Autodesk Fusion 360 part; units mm, degrees
(part 8 of 15)
  spline S16 degree 5 poles (-0.9615, -15.0052) (-0.9615, -15.0053) (-0.9615, -15.0055) (-0.9615, -15.0058) (-0.9616, -15.0063) (-0.9616, -15.0071) (-0.9616, -15.008) (-0.9617, -15.0091) (-0.9617, -15.0102) (-0.9618, -15.0115) (-0.9618, -15.0128) (-0.9619, -15.0143) (-0.9619, -15.0159) (-0.9619, -15.0176) (-0.962, -15.0194) (-0.962, -15.0213) (-0.962, -15.0234) (-0.9621, -15.0255) (-0.9621, -15.0277) (-0.9621, -15.0301) (-0.9621, -15.0325) (-0.9621, -15.0351) (-0.9621, -15.0377) (-0.9621, -15.0404) (-0.9621, -15.0433) (-0.9621, -15.0462) (-0.962, -15.0492) (-0.962, -15.0523) (-0.9619, -15.0555) (-0.9619, -15.0588) (-0.9618, -15.0622) (-0.9617, -15.0657) (-0.9616, -15.0693) (-0.9615, -15.0729) (-0.9614, -15.0767) (-0.9612, -15.0805) (-0.9611, -15.0844) (-0.9609, -15.0884) (-0.9607, -15.0925) (-0.9606, -15.0967) (-0.9603, -15.1009) (-0.9601, -15.1053) (-0.9599, -15.1097) (-0.9596, -15.1142) (-0.9594, -15.1187) (-0.9591, -15.1234) (-0.9588, -15.1281) (-0.9585, -15.1329) (-0.9581, -15.1378) (-0.9578, -15.1427) (-0.9574, -15.1477) (-0.957, -15.1528) (-0.9566, -15.158) (-0.9562, -15.1633) (-0.9558, -15.1686) (-0.9553, -15.174) (-0.9548, -15.1794) (-0.9543, -15.1849) (-0.9538, -15.1905) (-0.9533, -15.1962) (-0.9527, -15.2019) (-0.9521, -15.2077) (-0.9515, -15.2136) (-0.9509, -15.2196) (-0.9503, -15.2256) (-0.9496, -15.2316) (-0.9489, -15.2378) (-0.9482, -15.244) (-0.9475, -15.2502) (-0.9467, -15.2565) (-0.946, -15.2629) (-0.9452, -15.2694) (-0.9444, -15.2759) (-0.9435, -15.2825) (-0.9427, -15.2891) (-0.9418, -15.2958) (-0.9408, -15.3025) (-0.9399, -15.3094) (-0.9389, -15.3162) (-0.938, -15.3232) (-0.937, -15.3301) (-0.9359, -15.3372) (-0.9349, -15.3443) (-0.9338, -15.3515) (-0.9327, -15.3587) (-0.9315, -15.3659) (-0.9304, -15.3733) (-0.9292, -15.3807) (-0.928, -15.3881) (-0.9267, -15.3956) (-0.9255, -15.4031) (-0.9242, -15.4107) (-0.9229, -15.4184) (-0.9215, -15.4261) (-0.9202, -15.4338) (-0.9188, -15.4417) (-0.9173, -15.4495) (-0.9159, -15.4574) (-0.9144, -15.4654) (-0.9129, -15.4734) (-0.9114, -15.4815) (-0.9098, -15.4896) (-0.9082, -15.4977) (-0.9066, -15.5059) (-0.905, -15.5142) (-0.9033, -15.5225) (-0.9016, -15.5309) (-0.8999, -15.5393) (-0.8981, -15.5477) (-0.8963, -15.5562) (-0.8945, -15.5648) (-0.8927, -15.5733) (-0.8908, -15.582) (-0.8889, -15.5907) (-0.887, -15.5994) (-0.885, -15.6081) (-0.883, -15.617) (-0.881, -15.6258) (-0.879, -15.6347) (-0.8769, -15.6437) (-0.8748, -15.6527) (-0.8726, -15.6617) (-0.8705, -15.6708) (-0.8683, -15.6799) (-0.866, -15.689) (-0.8638, -15.6982) (-0.8615, -15.7075) (-0.8592, -15.7168) (-0.8568, -15.7261) (-0.8544, -15.7354) (-0.852, -15.7448) (-0.8496, -15.7543) (-0.8471, -15.7638) (-0.8446, -15.7733) (-0.8421, -15.7829) (-0.8395, -15.7925) (-0.8369, -15.8021) (-0.8343, -15.8118) (-0.8316, -15.8215) (-0.8289, -15.8313) (-0.8262, -15.841) (-0.8235, -15.8509) (-0.8207, -15.8607) (-0.8178, -15.8706) (-0.815, -15.8806) (-0.8121, -15.8906) (-0.8092, -15.9006) (-0.8063, -15.9106) (-0.8033, -15.9207) (-0.8003, -15.9308) (-0.7972, -15.941) (-0.7941, -15.9512) (-0.791, -15.9614) (-0.7879, -15.9716) (-0.7847, -15.9819) (-0.7815, -15.9923) (-0.7783, -16.0026) (-0.775, -16.013) (-0.7717, -16.0234) (-0.7683, -16.0339) (-0.765, -16.0444) (-0.7616, -16.0549) (-0.7581, -16.0655) (-0.7547, -16.0761) (-0.7512, -16.0867) (-0.7476, -16.0973) (-0.744, -16.108) (-0.7404, -16.1187) (-0.7368, -16.1295) (-0.7331, -16.1402) (-0.7294, -16.151) (-0.7257, -16.1619) (-0.7219, -16.1727) (-0.7181, -16.1836) (-0.7143, -16.1946) (-0.7104, -16.2055) (-0.7065, -16.2165) (-0.7025, -16.2275) (-0.6986, -16.2385) (-0.6946, -16.2496) (-0.6905, -16.2607) (-0.6864, -16.2718) (-0.6823, -16.283) (-0.6782, -16.2942) (-0.674, -16.3054) (-0.6698, -16.3166) (-0.6655, -16.3279) (-0.6612, -16.3391) (-0.6569, -16.3505) (-0.6526, -16.3618) (-0.6482, -16.3732) (-0.6438, -16.3846) (-0.6393, -16.396) (-0.6348, -16.4074) (-0.6303, -16.4189) (-0.6257, -16.4304) (-0.6211, -16.4419) (-0.6165, -16.4535) (-0.6118, -16.465) (-0.6071, -16.4766) (-0.6024, -16.4882) (-0.5976, -16.4999) (-0.5928, -16.5116) (-0.588, -16.5233) (-0.5831, -16.535) (-0.5782, -16.5467) (-0.5732, -16.5585) (-0.5683, -16.5703) (-0.5632, -16.5821) (-0.5582, -16.5939) (-0.5531, -16.6057) (-0.548, -16.6176) (-0.5428, -16.6295) (-0.5376, -16.6414) (-0.5324, -16.6534) (-0.5271, -16.6653) (-0.5218, -16.6773) (-0.5165, -16.6893) (-0.5111, -16.7014) (-0.5057, -16.7134) (-0.5003, -16.7255) (-0.4948, -16.7376) (-0.4893, -16.7497) (-0.4837, -16.7618) (-0.4782, -16.774) (-0.4725, -16.7861) (-0.4669, -16.7983) (-0.4612, -16.8105) (-0.4555, -16.8228) (-0.4497, -16.835) (-0.4439, -16.8473) (-0.4381, -16.8596) (-0.4322, -16.8719) (-0.4263, -16.8842) (-0.4203, -16.8965) (-0.4144, -16.9089) (-0.4084, -16.9213) (-0.4023, -16.9337) (-0.3962, -16.9461) (-0.3901, -16.9585) (-0.3839, -16.971) (-0.379, -16.981) (-0.3753, -16.9884) (-0.3728, -16.9934) (-0.3715, -16.9959) knots 0 0 0 0 0 0 0.00416667 0.00833333 0.0125 0.01666667 0.02083333 0.025 0.02916667 0.03333333 0.0375 0.04166667 0.04583333 0.05 0.05416667 0.05833333 0.0625 0.06666667 0.07083333 0.075 0.07916667 0.08333333 0.0875 0.09166667 0.09583333 0.1 0.10416667 0.10833333 0.1125 0.11666667 0.12083333 0.125 0.12916667 0.13333333 0.1375 0.14166667 0.14583333 0.15 0.15416667 0.15833333 0.1625 0.16666667 0.17083333 0.175 0.17916667 0.18333333 0.1875 0.19166667 0.19583333 0.2 0.20416667 0.20833333 0.2125 0.21666667 0.22083333 0.225 0.22916667 0.23333333 0.2375 0.24166667 0.24583333 0.25 0.25416667 0.25833333 0.2625 0.26666667 0.27083333 0.275 0.27916667 0.28333333 0.2875 0.29166667 0.29583333 0.3 0.30416667 0.30833333 0.3125 0.31666667 0.32083333 0.325 0.32916667 0.33333333 0.3375 0.34166667 0.34583333 0.35 0.35416667 0.35833333 0.3625 0.36666667 0.37083333 0.375 0.37916667 0.38333333 0.3875 0.39166667 0.39583333 0.4 0.40416667 0.40833333 0.4125 0.41666667 0.42083333 0.425 0.42916667 0.43333333 0.4375 0.44166667 0.44583333 0.45 0.45416667 0.45833333 0.4625 0.46666667 0.47083333 0.475 0.47916667 0.48333333 0.4875 0.49166667 0.49583333 0.5 0.50416667 0.50833333 0.5125 0.51666667 0.52083333 0.525 0.52916667 0.53333333 0.5375 0.54166667 0.54583333 0.55 0.55416667 0.55833333 0.5625 0.56666667 0.57083333 0.575 0.57916667 0.58333333 0.5875 0.59166667 0.59583333 0.6 0.60416667 0.60833333 0.6125 0.61666667 0.62083333 0.625 0.62916667 0.63333333 0.6375 0.64166667 0.64583333 0.65 0.65416667 0.65833333 0.6625 0.66666667 0.67083333 0.675 0.67916667 0.68333333 0.6875 0.69166667 0.69583333 0.7 0.70416667 0.70833333 0.7125 0.71666667 0.72083333 0.725 0.72916667 0.73333333 0.7375 0.74166667 0.74583333 0.75 0.75416667 0.75833333 0.7625 0.76666667 0.77083333 0.775 0.77916667 0.78333333 0.7875 0.79166667 0.79583333 0.8 0.80416667 0.80833333 0.8125 0.81666667 0.82083333 0.825 0.82916667 0.83333333 0.8375 0.84166667 0.84583333 0.85 0.85416667 0.85833333 0.8625 0.86666667 0.87083333 0.875 0.87916667 0.88333333 0.8875 0.89166667 0.89583333 0.9 0.90416667 0.90833333 0.9125 0.91666667 0.92083333 0.925 0.92916667 0.93333333 0.9375 0.94166667 0.94583333 0.95 0.95416667 0.95833333 0.9625 0.96666667 0.97083333 0.975 0.97916667 0.98333333 0.9875 0.99166667 0.99583333 1 1 1 1 1 1
  arc A17 (-0.3715, -16.9959) -> (0.3715, -16.9959) centre (0, 0) ccw
  spline S17 degree 5 poles (0.3715, -16.9959) (0.3728, -16.9934) (0.3753, -16.9884) (0.379, -16.981) (0.3839, -16.971) (0.3901, -16.9585) (0.3962, -16.9461) (0.4023, -16.9337) (0.4084, -16.9213) (0.4144, -16.9089) (0.4203, -16.8965) (0.4263, -16.8842) (0.4322, -16.8719) (0.4381, -16.8596) (0.4439, -16.8473) (0.4497, -16.835) (0.4555, -16.8228) (0.4612, -16.8105) (0.4669, -16.7983) (0.4725, -16.7861) (0.4782, -16.774) (0.4837, -16.7618) (0.4893, -16.7497) (0.4948, -16.7376) (0.5003, -16.7255) (0.5057, -16.7134) (0.5111, -16.7014) (0.5165, -16.6893) (0.5218, -16.6773) (0.5271, -16.6653) (0.5324, -16.6534) (0.5376, -16.6414) (0.5428, -16.6295) (0.548, -16.6176) (0.5531, -16.6057) (0.5582, -16.5939) (0.5632, -16.5821) (0.5683, -16.5703) (0.5732, -16.5585) (0.5782, -16.5467) (0.5831, -16.535) (0.588, -16.5233) (0.5928, -16.5116) (0.5976, -16.4999) (0.6024, -16.4882) (0.6071, -16.4766) (0.6118, -16.465) (0.6165, -16.4535) (0.6211, -16.4419) (0.6257, -16.4304) (0.6303, -16.4189) (0.6348, -16.4074) (0.6393, -16.396) (0.6438, -16.3846) (0.6482, -16.3732) (0.6526, -16.3618) (0.6569, -16.3505) (0.6612, -16.3391) (0.6655, -16.3279) (0.6698, -16.3166) (0.674, -16.3054) (0.6782, -16.2942) (0.6823, -16.283) (0.6864, -16.2718) (0.6905, -16.2607) (0.6946, -16.2496) (0.6986, -16.2385) (0.7025, -16.2275) (0.7065, -16.2165) (0.7104, -16.2055) (0.7143, -16.1946) (0.7181, -16.1836) (0.7219, -16.1727) (0.7257, -16.1619) (0.7294, -16.151) (0.7331, -16.1402) (0.7368, -16.1295) (0.7404, -16.1187) (0.744, -16.108) (0.7476, -16.0973) (0.7512, -16.0867) (0.7547, -16.0761) (0.7581, -16.0655) (0.7616, -16.0549) (0.765, -16.0444) (0.7683, -16.0339) (0.7717, -16.0234) (0.775, -16.013) (0.7783, -16.0026) (0.7815, -15.9923) (0.7847, -15.9819) (0.7879, -15.9716) (0.791, -15.9614) (0.7941, -15.9512) (0.7972, -15.941) (0.8003, -15.9308) (0.8033, -15.9207) (0.8063, -15.9106) (0.8092, -15.9006) (0.8121, -15.8906) (0.815, -15.8806) (0.8178, -15.8706) (0.8207, -15.8607) (0.8235, -15.8509) (0.8262, -15.841) (0.8289, -15.8313) (0.8316, -15.8215) (0.8343, -15.8118) (0.8369, -15.8021) (0.8395, -15.7925) (0.8421, -15.7829) (0.8446, -15.7733) (0.8471, -15.7638) (0.8496, -15.7543) (0.852, -15.7448) (0.8544, -15.7354) (0.8568, -15.7261) (0.8592, -15.7168) (0.8615, -15.7075) (0.8638, -15.6982) (0.866, -15.689) (0.8683, -15.6799) (0.8705, -15.6708) (0.8726, -15.6617) (0.8748, -15.6527) (0.8769, -15.6437) (0.879, -15.6347) (0.881, -15.6258) (0.883, -15.617) (0.885, -15.6081) (0.887, -15.5994) (0.8889, -15.5907) (0.8908, -15.582) (0.8927, -15.5733) (0.8945, -15.5648) (0.8963, -15.5562) (0.8981, -15.5477) (0.8999, -15.5393) (0.9016, -15.5309) (0.9033, -15.5225) (0.905, -15.5142) (0.9066, -15.5059) (0.9082, -15.4977) (0.9098, -15.4896) (0.9114, -15.4815) (0.9129, -15.4734) (0.9144, -15.4654) (0.9159, -15.4574) (0.9173, -15.4495) (0.9188, -15.4417) (0.9202, -15.4338) (0.9215, -15.4261) (0.9229, -15.4184) (0.9242, -15.4107) (0.9255, -15.4031) (0.9267, -15.3956) (0.928, -15.3881) (0.9292, -15.3807) (0.9304, -15.3733) (0.9315, -15.3659) (0.9327, -15.3587) (0.9338, -15.3515) (0.9349, -15.3443) (0.9359, -15.3372) (0.937, -15.3301) (0.938, -15.3232) (0.9389, -15.3162) (0.9399, -15.3094) (0.9408, -15.3025) (0.9418, -15.2958) (0.9427, -15.2891) (0.9435, -15.2825) (0.9444, -15.2759) (0.9452, -15.2694) (0.946, -15.2629) (0.9467, -15.2565) (0.9475, -15.2502) (0.9482, -15.244) (0.9489, -15.2378) (0.9496, -15.2316) (0.9503, -15.2256) (0.9509, -15.2196) (0.9515, -15.2136) (0.9521, -15.2077) (0.9527, -15.2019) (0.9533, -15.1962) (0.9538, -15.1905) (0.9543, -15.1849) (0.9548, -15.1794) (0.9553, -15.174) (0.9558, -15.1686) (0.9562, -15.1633) (0.9566, -15.158) (0.957, -15.1528) (0.9574, -15.1477) (0.9578, -15.1427) (0.9581, -15.1378) (0.9585, -15.1329) (0.9588, -15.1281) (0.9591, -15.1234) (0.9594, -15.1187) (0.9596, -15.1142) (0.9599, -15.1097) (0.9601, -15.1053) (0.9603, -15.1009) (0.9606, -15.0967) (0.9607, -15.0925) (0.9609, -15.0884) (0.9611, -15.0844) (0.9612, -15.0805) (0.9614, -15.0767) (0.9615, -15.0729) (0.9616, -15.0693) (0.9617, -15.0657) (0.9618, -15.0622) (0.9619, -15.0588) (0.9619, -15.0555) (0.962, -15.0523) (0.962, -15.0492) (0.9621, -15.0462) (0.9621, -15.0433) (0.9621, -15.0404) (0.9621, -15.0377) (0.9621, -15.0351) (0.9621, -15.0325) (0.9621, -15.0301) (0.9621, -15.0277) (0.9621, -15.0255) (0.962, -15.0234) (0.962, -15.0213) (0.962, -15.0194) (0.9619, -15.0176) (0.9619, -15.0159) (0.9619, -15.0143) (0.9618, -15.0128) (0.9618, -15.0115) (0.9617, -15.0102) (0.9617, -15.0091) (0.9616, -15.008) (0.9616, -15.0071) (0.9616, -15.0063) (0.9615, -15.0058) (0.9615, -15.0055) (0.9615, -15.0053) (0.9615, -15.0052) knots -1 -1 -1 -1 -1 -1 -0.99583333 -0.99166667 -0.9875 -0.98333333 -0.97916667 -0.975 -0.97083333 -0.96666667 -0.9625 -0.95833333 -0.95416667 -0.95 -0.94583333 -0.94166667 -0.9375 -0.93333333 -0.92916667 -0.925 -0.92083333 -0.91666667 -0.9125 -0.90833333 -0.90416667 -0.9 -0.89583333 -0.89166667 -0.8875 -0.88333333 -0.87916667 -0.875 -0.87083333 -0.86666667 -0.8625 -0.85833333 -0.85416667 -0.85 -0.84583333 -0.84166667 -0.8375 -0.83333333 -0.82916667 -0.825 -0.82083333 -0.81666667 -0.8125 -0.80833333 -0.80416667 -0.8 -0.79583333 -0.79166667 -0.7875 -0.78333333 -0.77916667 -0.775 -0.77083333 -0.76666667 -0.7625 -0.75833333 -0.75416667 -0.75 -0.74583333 -0.74166667 -0.7375 -0.73333333 -0.72916667 -0.725 -0.72083333 -0.71666667 -0.7125 -0.70833333 -0.70416667 -0.7 -0.69583333 -0.69166667 -0.6875 -0.68333333 -0.67916667 -0.675 -0.67083333 -0.66666667 -0.6625 -0.65833333 -0.65416667 -0.65 -0.64583333 -0.64166667 -0.6375 -0.63333333 -0.62916667 -0.625 -0.62083333 -0.61666667 -0.6125 -0.60833333 -0.60416667 -0.6 -0.59583333 -0.59166667 -0.5875 -0.58333333 -0.57916667 -0.575 -0.57083333 -0.56666667 -0.5625 -0.55833333 -0.55416667 -0.55 -0.54583333 -0.54166667 -0.5375 -0.53333333 -0.52916667 -0.525 -0.52083333 -0.51666667 -0.5125 -0.50833333 -0.50416667 -0.5 -0.49583333 -0.49166667 -0.4875 -0.48333333 -0.47916667 -0.475 -0.47083333 -0.46666667 -0.4625 -0.45833333 -0.45416667 -0.45 -0.44583333 -0.44166667 -0.4375 -0.43333333 -0.42916667 -0.425 -0.42083333 -0.41666667 -0.4125 -0.40833333 -0.40416667 -0.4 -0.39583333 -0.39166667 -0.3875 -0.38333333 -0.37916667 -0.375 -0.37083333 -0.36666667 -0.3625 -0.35833333 -0.35416667 -0.35 -0.34583333 -0.34166667 -0.3375 -0.33333333 -0.32916667 -0.325 -0.32083333 -0.31666667 -0.3125 -0.30833333 -0.30416667 -0.3 -0.29583333 -0.29166667 -0.2875 -0.28333333 -0.27916667 -0.275 -0.27083333 -0.26666667 -0.2625 -0.25833333 -0.25416667 -0.25 -0.24583333 -0.24166667 -0.2375 -0.23333333 -0.22916667 -0.225 -0.22083333 -0.21666667 -0.2125 -0.20833333 -0.20416667 -0.2 -0.19583333 -0.19166667 -0.1875 -0.18333333 -0.17916667 -0.175 -0.17083333 -0.16666667 -0.1625 -0.15833333 -0.15416667 -0.15 -0.14583333 -0.14166667 -0.1375 -0.13333333 -0.12916667 -0.125 -0.12083333 -0.11666667 -0.1125 -0.10833333 -0.10416667 -0.1 -0.09583333 -0.09166667 -0.0875 -0.08333333 -0.07916667 -0.075 -0.07083333 -0.06666667 -0.0625 -0.05833333 -0.05416667 -0.05 -0.04583333 -0.04166667 -0.0375 -0.03333333 -0.02916667 -0.025 -0.02083333 -0.01666667 -0.0125 -0.00833333 -0.00416667 0 0 0 0 0 0
  line L34 (0.9615, -15.0052) -> (0.9615, -15.0043)
  line L35 (0.9615, -15.0043) -> (0.9432, -14.7198)
  arc A18 (0.9432, -14.7198) -> (1.9466, -14.621) centre (0, 0) ccw
  line L36 (1.9466, -14.621) -> (1.9842, -14.9036)
  line L37 (1.9842, -14.9036) -> (1.9843, -14.9044)
  spline S18 degree 5 poles (1.9843, -14.9044) (1.9843, -14.9045) (1.9844, -14.9047) (1.9844, -14.9051) (1.9845, -14.9056) (1.9846, -14.9064) (1.9848, -14.9073) (1.9849, -14.9083) (1.9851, -14.9094) (1.9853, -14.9106) (1.9855, -14.912) (1.9858, -14.9135) (1.986, -14.915) (1.9863, -14.9167) (1.9866, -14.9185) (1.987, -14.9204) (1.9874, -14.9224) (1.9877, -14.9245) (1.9882, -14.9267) (1.9886, -14.929) (1.9891, -14.9314) (1.9896, -14.9339) (1.9901, -14.9365) (1.9906, -14.9391) (1.9912, -14.9419) (1.9918, -14.9448) (1.9924, -14.9477) (1.9931, -14.9508) (1.9937, -14.9539) (1.9945, -14.9571) (1.9952, -14.9605) (1.996, -14.9639) (1.9968, -14.9673) (1.9976, -14.9709) (1.9984, -14.9746) (1.9993, -14.9783) (2.0002, -14.9821) (2.0012, -14.986) (2.0021, -14.99) (2.0031, -14.994) (2.0042, -14.9981) (2.0052, -15.0023) (2.0063, -15.0066) (2.0074, -15.011) (2.0086, -15.0154) (2.0098, -15.0199) (2.011, -15.0245) (2.0122, -15.0291) (2.0135, -15.0338) (2.0148, -15.0386) (2.0161, -15.0435) (2.0175, -15.0484) (2.0189, -15.0534) (2.0204, -15.0584) (2.0218, -15.0636) (2.0233, -15.0688) (2.0249, -15.074) (2.0264, -15.0794) (2.028, -15.0847) (2.0297, -15.0902) (2.0313, -15.0957) (2.033, -15.1013) (2.0348, -15.1069) (2.0365, -15.1126) (2.0383, -15.1184) (2.0402, -15.1242) (2.042, -15.1301) (2.0439, -15.136) (2.0459, -15.142) (2.0478, -15.1481) (2.0499, -15.1542) (2.0519, -15.1604) (2.054, -15.1666) (2.0561, -15.1729) (2.0582, -15.1792) (2.0604, -15.1856) (2.0626, -15.1921) (2.0649, -15.1986) (2.0671, -15.2051) (2.0695, -15.2117) (2.0718, -15.2184) (2.0742, -15.2251) (2.0766, -15.2318) (2.0791, -15.2387) (2.0816, -15.2455) (2.0841, -15.2524) (2.0867, -15.2594) (2.0893, -15.2664) (2.0919, -15.2735) (2.0946, -15.2806) (2.0973, -15.2877) (2.1001, -15.2949) (2.1028, -15.3022) (2.1057, -15.3095) (2.1085, -15.3168) (2.1114, -15.3242) (2.1143, -15.3316) (2.1173, -15.3391) (2.1203, -15.3466) (2.1233, -15.3542) (2.1264, -15.3618) (2.1295, -15.3694) (2.1327, -15.3771) (2.1359, -15.3849) (2.1391, -15.3927) (2.1423, -15.4005) (2.1456, -15.4083) (2.149, -15.4162) (2.1523, -15.4242) (2.1558, -15.4322) (2.1592, -15.4402) (2.1627, -15.4483) (2.1662, -15.4564) (2.1698, -15.4645) (2.1734, -15.4727) (2.177, -15.4809) (2.1807, -15.4892) (2.1844, -15.4974) (2.1881, -15.5058) (2.1919, -15.5141) (2.1957, -15.5226) (2.1996, -15.531) (2.2035, -15.5395) (2.2074, -15.548) (2.2114, -15.5565) (2.2154, -15.5651) (2.2194, -15.5737) (2.2235, -15.5824) (2.2276, -15.5911) (2.2318, -15.5998) (2.236, -15.6085) (2.2402, -15.6173) (2.2445, -15.6261) (2.2488, -15.635) (2.2532, -15.6439) (2.2576, -15.6528) (2.262, -15.6617) (2.2665, -15.6707) (2.271, -15.6797) (2.2755, -15.6888) (2.2801, -15.6979) (2.2847, -15.707) (2.2894, -15.7161) (2.2941, -15.7253) (2.2988, -15.7344) (2.3036, -15.7437) (2.3084, -15.7529) (2.3132, -15.7622) (2.3181, -15.7715) (2.3231, -15.7808) (2.328, -15.7902) (2.333, -15.7996) (2.3381, -15.809) (2.3432, -15.8185) (2.3483, -15.8279) (2.3534, -15.8374) (2.3586, -15.847) (2.3639, -15.8565) (2.3692, -15.8661) (2.3745, -15.8757) (2.3798, -15.8853) (2.3852, -15.895) (2.3907, -15.9047) (2.3961, -15.9144) (2.4016, -15.9241) (2.4072, -15.9339) (2.4128, -15.9436) (2.4184, -15.9535) (2.4241, -15.9633) (2.4298, -15.9731) (2.4355, -15.983) (2.4413, -15.9929) (2.4471, -16.0028) (2.453, -16.0128) (2.4589, -16.0227) (2.4648, -16.0327) (2.4708, -16.0427) (2.4768, -16.0527) (2.4828, -16.0628) (2.4889, -16.0729) (2.4951, -16.083) (2.5012, -16.0931) (2.5074, -16.1032) (2.5137, -16.1134) (2.52, -16.1235) (2.5263, -16.1337) (2.5327, -16.144) (2.5391, -16.1542) (2.5455, -16.1645) (2.552, -16.1747) (2.5585, -16.185) (2.5651, -16.1953) (2.5717, -16.2057) (2.5783, -16.216) (2.585, -16.2264) (2.5917, -16.2368) (2.5985, -16.2472) (2.6053, -16.2576) (2.6121, -16.268) (2.619, -16.2785) (2.6259, -16.289) (2.6328, -16.2994) (2.6398, -16.3099) (2.6469, -16.3205) (2.6539, -16.331) (2.661, -16.3416) (2.6682, -16.3521) (2.6754, -16.3627) (2.6826, -16.3733) (2.6898, -16.3839) (2.6971, -16.3946) (2.7045, -16.4052) (2.7119, -16.4159) (2.7193, -16.4266) (2.7267, -16.4373) (2.7342, -16.448) (2.7418, -16.4587) (2.7494, -16.4694) (2.757, -16.4802) (2.7646, -16.4909) (2.7723, -16.5017) (2.78, -16.5125) (2.7878, -16.5233) (2.7956, -16.5341) (2.8035, -16.5449) (2.8114, -16.5558) (2.8193, -16.5666) (2.8272, -16.5775) (2.8352, -16.5884) (2.8433, -16.5993) (2.8514, -16.6102) (2.8595, -16.6211) (2.8676, -16.632) (2.8758, -16.6429) (2.8841, -16.6539) (2.8924, -16.6648) (2.9007, -16.6758) (2.909, -16.6868) (2.9174, -16.6978) (2.9258, -16.7088) (2.9343, -16.7198) (2.9411, -16.7286) (2.9462, -16.7352) (2.9497, -16.7396) (2.9514, -16.7418) knots 0 0 0 0 0 0 0.00416667 0.00833333 0.0125 0.01666667 0.02083333 0.025 0.02916667 0.03333333 0.0375 0.04166667 0.04583333 0.05 0.05416667 0.05833333 0.0625 0.06666667 0.07083333 0.075 0.07916667 0.08333333 0.0875 0.09166667 0.09583333 0.1 0.10416667 0.10833333 0.1125 0.11666667 0.12083333 0.125 0.12916667 0.13333333 0.1375 0.14166667 0.14583333 0.15 0.15416667 0.15833333 0.1625 0.16666667 0.17083333 0.175 0.17916667 0.18333333 0.1875 0.19166667 0.19583333 0.2 0.20416667 0.20833333 0.2125 0.21666667 0.22083333 0.225 0.22916667 0.23333333 0.2375 0.24166667 0.24583333 0.25 0.25416667 0.25833333 0.2625 0.26666667 0.27083333 0.275 0.27916667 0.28333333 0.2875 0.29166667 0.29583333 0.3 0.30416667 0.30833333 0.3125 0.31666667 0.32083333 0.325 0.32916667 0.33333333 0.3375 0.34166667 0.34583333 0.35 0.35416667 0.35833333 0.3625 0.36666667 0.37083333 0.375 0.37916667 0.38333333 0.3875 0.39166667 0.39583333 0.4 0.40416667 0.40833333 0.4125 0.41666667 0.42083333 0.425 0.42916667 0.43333333 0.4375 0.44166667 0.44583333 0.45 0.45416667 0.45833333 0.4625 0.46666667 0.47083333 0.475 0.47916667 0.48333333 0.4875 0.49166667 0.49583333 0.5 0.50416667 0.50833333 0.5125 0.51666667 0.52083333 0.525 0.52916667 0.53333333 0.5375 0.54166667 0.54583333 0.55 0.55416667 0.55833333 0.5625 0.56666667 0.57083333 0.575 0.57916667 0.58333333 0.5875 0.59166667 0.59583333 0.6 0.60416667 0.60833333 0.6125 0.61666667 0.62083333 0.625 0.62916667 0.63333333 0.6375 0.64166667 0.64583333 0.65 0.65416667 0.65833333 0.6625 0.66666667 0.67083333 0.675 0.67916667 0.68333333 0.6875 0.69166667 0.69583333 0.7 0.70416667 0.70833333 0.7125 0.71666667 0.72083333 0.725 0.72916667 0.73333333 0.7375 0.74166667 0.74583333 0.75 0.75416667 0.75833333 0.7625 0.76666667 0.77083333 0.775 0.77916667 0.78333333 0.7875 0.79166667 0.79583333 0.8 0.80416667 0.80833333 0.8125 0.81666667 0.82083333 0.825 0.82916667 0.83333333 0.8375 0.84166667 0.84583333 0.85 0.85416667 0.85833333 0.8625 0.86666667 0.87083333 0.875 0.87916667 0.88333333 0.8875 0.89166667 0.89583333 0.9 0.90416667 0.90833333 0.9125 0.91666667 0.92083333 0.925 0.92916667 0.93333333 0.9375 0.94166667 0.94583333 0.95 0.95416667 0.95833333 0.9625 0.96666667 0.97083333 0.975 0.97916667 0.98333333 0.9875 0.99166667 0.99583333 1 1 1 1 1 1
  arc A19 (2.9514, -16.7418) -> (3.6801, -16.5969) centre (0, 0) ccw
  spline S19 degree 5 poles (3.6801, -16.5969) (3.6808, -16.5942) (3.6823, -16.5888) (3.6845, -16.5807) (3.6874, -16.57) (3.691, -16.5566) (3.6946, -16.5432) (3.6982, -16.5298) (3.7017, -16.5165) (3.7052, -16.5032) (3.7086, -16.4899) (3.712, -16.4766) (3.7154, -16.4634) (3.7188, -16.4502) (3.7221, -16.437) (3.7254, -16.4238) (3.7287, -16.4107) (3.7319, -16.3976) (3.7351, -16.3845) (3.7383, -16.3714) (3.7414, -16.3584) (3.7445, -16.3454) (3.7476, -16.3324) (3.7506, -16.3194) (3.7536, -16.3065) (3.7566, -16.2936) (3.7596, -16.2807) (3.7625, -16.2679) (3.7654, -16.2551) (3.7683, -16.2423) (3.7711, -16.2295) (3.7739, -16.2168) (3.7766, -16.2041) (3.7794, -16.1914) (3.7821, -16.1788) (3.7848, -16.1661) (3.7874, -16.1536) (3.79, -16.141) (3.7926, -16.1285) (3.7952, -16.116) (3.7977, -16.1035) (3.8002, -16.0911) (3.8027, -16.0786) (3.8051, -16.0663) (3.8075, -16.0539) (3.8099, -16.0416) (3.8122, -16.0293) (3.8146, -16.017) (3.8168, -16.0048) (3.8191, -15.9926) (3.8213, -15.9805) (3.8235, -15.9683) (3.8257, -15.9562) (3.8279, -15.9441) (3.83, -15.9321) (3.8321, -15.9201) (3.8341, -15.9081) (3.8361, -15.8962) (3.8381, -15.8843) (3.8401, -15.8724) (3.8421, -15.8606) (3.844, -15.8488) (3.8459, -15.837) (3.8477, -15.8252) (3.8495, -15.8135) (3.8513, -15.8019) (3.8531, -15.7902) (3.8549, -15.7786) (3.8566, -15.7671) (3.8583, -15.7555) (3.8599, -15.744) (3.8616, -15.7326) (3.8632, -15.7211) (3.8648, -15.7097) (3.8663, -15.6984) (3.8678, -15.6871) (3.8693, -15.6758) (3.8708, -15.6645) (3.8723, -15.6533) (3.8737, -15.6422) (3.8751, -15.631) (3.8764, -15.6199) (3.8778, -15.6089) (3.8791, -15.5978) (3.8804, -15.5869) (3.8816, -15.5759) (3.8829, -15.565) (3.8841, -15.5541) (3.8853, -15.5433) (3.8864, -15.5325) (3.8876, -15.5218) (3.8887, -15.511) (3.8897, -15.5004) (3.8908, -15.4897) (3.8918, -15.4791) (3.8928, -15.4686) (3.8938, -15.4581) (3.8948, -15.4476) (3.8957, -15.4372) (3.8966, -15.4268) (3.8975, -15.4164) (3.8983, -15.4061) (3.8992, -15.3959) (3.9, -15.3857) (3.9008, -15.3755) (3.9015, -15.3653) (3.9023, -15.3553) (3.903, -15.3452) (3.9037, -15.3352) (3.9043, -15.3252) (3.905, -15.3153) (3.9056, -15.3054) (3.9062, -15.2956) (3.9068, -15.2858) (3.9073, -15.2761) (3.9079, -15.2664) (3.9084, -15.2568) (3.9089, -15.2471) (3.9093, -15.2376) (3.9098, -15.2281) (3.9102, -15.2186) (3.9106, -15.2092) (3.911, -15.1998) (3.9113, -15.1905) (3.9116, -15.1812) (3.912, -15.172) (3.9123, -15.1628) (3.9125, -15.1537) (3.9128, -15.1446) (3.913, -15.1356) (3.9132, -15.1266) (3.9134, -15.1177) (3.9136, -15.1088) (3.9137, -15.0999) (3.9139, -15.0912) (3.914, -15.0824) (3.9141, -15.0738) (3.9141, -15.0651) (3.9142, -15.0565) (3.9142, -15.048) (3.9143, -15.0396) (3.9143, -15.0311) (3.9142, -15.0228) (3.9142, -15.0145) (3.9141, -15.0062) (3.9141, -14.998) (3.914, -14.9898) (3.9139, -14.9817) (3.9138, -14.9737) (3.9136, -14.9657) (3.9135, -14.9578) (3.9133, -14.9499) (3.9131, -14.9421) (3.9129, -14.9343) (3.9127, -14.9266) (3.9125, -14.919) (3.9122, -14.9114) (3.912, -14.9038) (3.9117, -14.8964) (3.9114, -14.889) (3.9111, -14.8816) (3.9108, -14.8743) (3.9104, -14.8671) (3.9101, -14.8599) (3.9097, -14.8528) (3.9093, -14.8457) (3.909, -14.8388) (3.9086, -14.8318) (3.9081, -14.825) (3.9077, -14.8182) (3.9073, -14.8114) (3.9068, -14.8047) (3.9064, -14.7981) (3.9059, -14.7916) (3.9054, -14.7851) (3.905, -14.7787) (3.9045, -14.7723) (3.904, -14.7661) (3.9034, -14.7598) (3.9029, -14.7537) (3.9024, -14.7476) (3.9018, -14.7416) (3.9013, -14.7357) (3.9007, -14.7298) (3.9002, -14.724) (3.8996, -14.7182) (3.899, -14.7126) (3.8984, -14.707) (3.8979, -14.7015) (3.8973, -14.696) (3.8967, -14.6907) (3.8961, -14.6854) (3.8954, -14.6801) (3.8948, -14.675) (3.8942, -14.6699) (3.8936, -14.6649) (3.893, -14.66) (3.8923, -14.6551) (3.8917, -14.6504) (3.8911, -14.6457) (3.8905, -14.6411) (3.8898, -14.6365) (3.8892, -14.6321) (3.8886, -14.6277) (3.8879, -14.6234) (3.8873, -14.6192) (3.8867, -14.6151) (3.8861, -14.6111) (3.8854, -14.6071) (3.8848, -14.6032) (3.8842, -14.5994) (3.8836, -14.5957) (3.883, -14.5921) (3.8824, -14.5886) (3.8818, -14.5852) (3.8812, -14.5818) (3.8806, -14.5786) (3.8801, -14.5754) (3.8795, -14.5724) (3.8789, -14.5694) (3.8784, -14.5665) (3.8779, -14.5637) (3.8773, -14.5611) (3.8768, -14.5585) (3.8763, -14.556) (3.8758, -14.5536) (3.8754, -14.5513) (3.8749, -14.5491) (3.8745, -14.547) (3.874, -14.545) (3.8736, -14.5432) (3.8733, -14.5414) (3.8729, -14.5397) (3.8725, -14.5382) (3.8722, -14.5367) (3.8719, -14.5354) (3.8716, -14.5342) (3.8713, -14.533) (3.8711, -14.532) (3.8709, -14.5312) (3.8707, -14.5304) (3.8706, -14.5299) (3.8705, -14.5296) (3.8704, -14.5294) (3.8704, -14.5293) knots -1 -1 -1 -1 -1 -1 -0.99583333 -0.99166667 -0.9875 -0.98333333 -0.97916667 -0.975 -0.97083333 -0.96666667 -0.9625 -0.95833333 -0.95416667 -0.95 -0.94583333 -0.94166667 -0.9375 -0.93333333 -0.92916667 -0.925 -0.92083333 -0.91666667 -0.9125 -0.90833333 -0.90416667 -0.9 -0.89583333 -0.89166667 -0.8875 -0.88333333 -0.87916667 -0.875 -0.87083333 -0.86666667 -0.8625 -0.85833333 -0.85416667 -0.85 -0.84583333 -0.84166667 -0.8375 -0.83333333 -0.82916667 -0.825 -0.82083333 -0.81666667 -0.8125 -0.80833333 -0.80416667 -0.8 -0.79583333 -0.79166667 -0.7875 -0.78333333 -0.77916667 -0.775 -0.77083333 -0.76666667 -0.7625 -0.75833333 -0.75416667 -0.75 -0.74583333 -0.74166667 -0.7375 -0.73333333 -0.72916667 -0.725 -0.72083333 -0.71666667 -0.7125 -0.70833333 -0.70416667 -0.7 -0.69583333 -0.69166667 -0.6875 -0.68333333 -0.67916667 -0.675 -0.67083333 -0.66666667 -0.6625 -0.65833333 -0.65416667 -0.65 -0.64583333 -0.64166667 -0.6375 -0.63333333 -0.62916667 -0.625 -0.62083333 -0.61666667 -0.6125 -0.60833333 -0.60416667 -0.6 -0.59583333 -0.59166667 -0.5875 -0.58333333 -0.57916667 -0.575 -0.57083333 -0.56666667 -0.5625 -0.55833333 -0.55416667 -0.55 -0.54583333 -0.54166667 -0.5375 -0.53333333 -0.52916667 -0.525 -0.52083333 -0.51666667 -0.5125 -0.50833333 -0.50416667 -0.5 -0.49583333 -0.49166667 -0.4875 -0.48333333 -0.47916667 -0.475 -0.47083333 -0.46666667 -0.4625 -0.45833333 -0.45416667 -0.45 -0.44583333 -0.44166667 -0.4375 -0.43333333 -0.42916667 -0.425 -0.42083333 -0.41666667 -0.4125 -0.40833333 -0.40416667 -0.4 -0.39583333 -0.39166667 -0.3875 -0.38333333 -0.37916667 -0.375 -0.37083333 -0.36666667 -0.3625 -0.35833333 -0.35416667 -0.35 -0.34583333 -0.34166667 -0.3375 -0.33333333 -0.32916667 -0.325 -0.32083333 -0.31666667 -0.3125 -0.30833333 -0.30416667 -0.3 -0.29583333 -0.29166667 -0.2875 -0.28333333 -0.27916667 -0.275 -0.27083333 -0.26666667 -0.2625 -0.25833333 -0.25416667 -0.25 -0.24583333 -0.24166667 -0.2375 -0.23333333 -0.22916667 -0.225 -0.22083333 -0.21666667 -0.2125 -0.20833333 -0.20416667 -0.2 -0.19583333 -0.19166667 -0.1875 -0.18333333 -0.17916667 -0.175 -0.17083333 -0.16666667 -0.1625 -0.15833333 -0.15416667 -0.15 -0.14583333 -0.14166667 -0.1375 -0.13333333 -0.12916667 -0.125 -0.12083333 -0.11666667 -0.1125 -0.10833333 -0.10416667 -0.1 -0.09583333 -0.09166667 -0.0875 -0.08333333 -0.07916667 -0.075 -0.07083333 -0.06666667 -0.0625 -0.05833333 -0.05416667 -0.05 -0.04583333 -0.04166667 -0.0375 -0.03333333 -0.02916667 -0.025 -0.02083333 -0.01666667 -0.0125 -0.00833333 -0.00416667 0 0 0 0 0 0
  line L38 (3.8704, -14.5293) -> (3.8702, -14.5284)
  line L39 (3.8702, -14.5284) -> (3.7968, -14.253)
  arc A20 (3.7968, -14.253) -> (4.7616, -13.9603) centre (0, 0) ccw
  line L40 (4.7616, -13.9603) -> (4.8536, -14.2301)
  line L41 (4.8536, -14.2301) -> (4.8539, -14.2309)
  spline S20 degree 5 poles (4.8539, -14.2309) (4.8539, -14.231) (4.854, -14.2312) (4.8541, -14.2315) (4.8543, -14.232) (4.8546, -14.2328) (4.8549, -14.2336) (4.8552, -14.2346) (4.8556, -14.2356) (4.8561, -14.2368) (4.8566, -14.2381) (4.8571, -14.2395) (4.8577, -14.241) (4.8583, -14.2426) (4.8589, -14.2443) (4.8596, -14.2461) (4.8604, -14.2479) (4.8612, -14.2499) (4.862, -14.252) (4.8629, -14.2542) (4.8638, -14.2564) (4.8648, -14.2588) (4.8658, -14.2612) (4.8669, -14.2637) (4.868, -14.2663) (4.8691, -14.269) (4.8703, -14.2718) (4.8715, -14.2747) (4.8728, -14.2776) (4.8741, -14.2807) (4.8755, -14.2838) (4.8769, -14.2869) (4.8784, -14.2902) (4.8799, -14.2935) (4.8814, -14.2969) (4.883, -14.3004) (4.8846, -14.304) (4.8863, -14.3076) (4.888, -14.3113) (4.8898, -14.3151) (4.8916, -14.319) (4.8935, -14.3229) (4.8954, -14.3269) (4.8973, -14.3309) (4.8993, -14.335) (4.9014, -14.3392) (4.9035, -14.3435) (4.9056, -14.3478) (4.9078, -14.3521) (4.91, -14.3566) (4.9122, -14.3611) (4.9145, -14.3656) (4.9169, -14.3703) (4.9193, -14.375) (4.9217, -14.3797) (4.9242, -14.3845) (4.9268, -14.3894) (4.9293, -14.3943) (4.932, -14.3992) (4.9346, -14.4043) (4.9373, -14.4094) (4.9401, -14.4145) (4.9429, -14.4197) (4.9457, -14.4249) (4.9486, -14.4302) (4.9516, -14.4356) (4.9545, -14.441) (4.9576, -14.4465) (4.9606, -14.452) (4.9637, -14.4575) (4.9669, -14.4631) (4.9701, -14.4688) (4.9734, -14.4745) (4.9766, -14.4802) (4.98, -14.486) (4.9834, -14.4919) (4.9868, -14.4978) (4.9903, -14.5037) (4.9938, -14.5097) (4.9974, -14.5157) (5.001, -14.5218) (5.0046, -14.5279) (5.0083, -14.534) (5.0121, -14.5402) (5.0158, -14.5465) (5.0197, -14.5528) (5.0235, -14.5591) (5.0275, -14.5655) (5.0314, -14.5719) (5.0354, -14.5783) (5.0395, -14.5848) (5.0436, -14.5913) (5.0477, -14.5979) (5.0519, -14.6045) (5.0562, -14.6111) (5.0604, -14.6178) (5.0648, -14.6245) (5.0691, -14.6313) (5.0735, -14.6381) (5.078, -14.6449) (5.0825, -14.6518) (5.087, -14.6587) (5.0916, -14.6656) (5.0963, -14.6726) (5.1009, -14.6796) (5.1057, -14.6866) (5.1104, -14.6937) (5.1152, -14.7008) (5.1201, -14.7079) (5.125, -14.7151) (5.1299, -14.7223) (5.1349, -14.7295) (5.14, -14.7368) (5.145, -14.7441) (5.1502, -14.7514) (5.1553, -14.7587) (5.1605, -14.7661) (5.1658, -14.7735) (5.1711, -14.781) (5.1764, -14.7884) (5.1818, -14.7959) (5.1873, -14.8035) (5.1927, -14.811) (5.1982, -14.8186) (5.2038, -14.8262) (5.2094, -14.8338) (5.2151, -14.8415) (5.2208, -14.8492) (5.2265, -14.8569) (5.2323, -14.8646) (5.2381, -14.8724) (5.244, -14.8802) (5.2499, -14.888) (5.2559, -14.8959) (5.2619, -14.9037) (5.2679, -14.9116) (5.274, -14.9195) (5.2801, -14.9275) (5.2863, -14.9354) (5.2925, -14.9434) (5.2988, -14.9514) (5.3051, -14.9594) (5.3114, -14.9675) (5.3178, -14.9755) (5.3243, -14.9836) (5.3308, -14.9918) (5.3373, -14.9999) (5.3439, -15.008) (5.3505, -15.0162) (5.3571, -15.0244) (5.3638, -15.0326) (5.3706, -15.0409) (5.3773, -15.0491) (5.3842, -15.0574) (5.391, -15.0657) (5.398, -15.074) (5.4049, -15.0823) (5.4119, -15.0907) (5.419, -15.099) (5.426, -15.1074) (5.4332, -15.1158) (5.4403, -15.1242) (5.4476, -15.1327) (5.4548, -15.1411) (5.4621, -15.1496) (5.4695, -15.1581) (5.4769, -15.1666) (5.4843, -15.1751) (5.4918, -15.1836) (5.4993, -15.1922) (5.5068, -15.2008) (5.5144, -15.2093) (5.5221, -15.2179) (5.5298, -15.2265) (5.5375, -15.2352) (5.5453, -15.2438) (5.5531, -15.2524) (5.5609, -15.2611) (5.5688, -15.2698) (5.5768, -15.2785) (5.5848, -15.2872) (5.5928, -15.2959) (5.6008, -15.3046) (5.609, -15.3134) (5.6171, -15.3221) (5.6253, -15.3309) (5.6335, -15.3397) (5.6418, -15.3484) (5.6501, -15.3572) (5.6585, -15.3661) (5.6669, -15.3749) (5.6753, -15.3837) (5.6838, -15.3926) (5.6924, -15.4014) (5.7009, -15.4103) (5.7096, -15.4192) (5.7182, -15.428) (5.7269, -15.4369) (5.7356, -15.4458) (5.7444, -15.4548) (5.7532, -15.4637) (5.7621, -15.4726) (5.771, -15.4816) (5.78, -15.4905) (5.789, -15.4995) (5.798, -15.5084) (5.8071, -15.5174) (5.8162, -15.5264) (5.8253, -15.5354) (5.8345, -15.5444) (5.8437, -15.5534) (5.853, -15.5624) (5.8623, -15.5714) (5.8717, -15.5804) (5.8811, -15.5895) (5.8905, -15.5985) (5.9, -15.6075) (5.9096, -15.6166) (5.9191, -15.6256) (5.9287, -15.6347) (5.9384, -15.6438) (5.9481, -15.6529) (5.9578, -15.6619) (5.9676, -15.671) (5.9774, -15.6801) (5.9872, -15.6892) (5.9971, -15.6983) (6.007, -15.7074) (6.017, -15.7165) (6.027, -15.7256) (6.0371, -15.7347) (6.0472, -15.7439) (6.0573, -15.753) (6.0675, -15.7621) (6.0777, -15.7712) (6.0879, -15.7804) (6.0982, -15.7895) (6.1086, -15.7986) (6.1189, -15.8078) (6.1293, -15.8169) (6.1398, -15.8261) (6.1482, -15.8334) (6.1545, -15.8389) (6.1587, -15.8425) (6.1608, -15.8444) knots 0 0 0 0 0 0 0.00416667 0.00833333 0.0125 0.01666667 0.02083333 0.025 0.02916667 0.03333333 0.0375 0.04166667 0.04583333 0.05 0.05416667 0.05833333 0.0625 0.06666667 0.07083333 0.075 0.07916667 0.08333333 0.0875 0.09166667 0.09583333 0.1 0.10416667 0.10833333 0.1125 0.11666667 0.12083333 0.125 0.12916667 0.13333333 0.1375 0.14166667 0.14583333 0.15 0.15416667 0.15833333 0.1625 0.16666667 0.17083333 0.175 0.17916667 0.18333333 0.1875 0.19166667 0.19583333 0.2 0.20416667 0.20833333 0.2125 0.21666667 0.22083333 0.225 0.22916667 0.23333333 0.2375 0.24166667 0.24583333 0.25 0.25416667 0.25833333 0.2625 0.26666667 0.27083333 0.275 0.27916667 0.28333333 0.2875 0.29166667 0.29583333 0.3 0.30416667 0.30833333 0.3125 0.31666667 0.32083333 0.325 0.32916667 0.33333333 0.3375 0.34166667 0.34583333 0.35 0.35416667 0.35833333 0.3625 0.36666667 0.37083333 0.375 0.37916667 0.38333333 0.3875 0.39166667 0.39583333 0.4 0.40416667 0.40833333 0.4125 0.41666667 0.42083333 0.425 0.42916667 0.43333333 0.4375 0.44166667 0.44583333 0.45 0.45416667 0.45833333 0.4625 0.46666667 0.47083333 0.475 0.47916667 0.48333333 0.4875 0.49166667 0.49583333 0.5 0.50416667 0.50833333 0.5125 0.51666667 0.52083333 0.525 0.52916667 0.53333333 0.5375 0.54166667 0.54583333 0.55 0.55416667 0.55833333 0.5625 0.56666667 0.57083333 0.575 0.57916667 0.58333333 0.5875 0.59166667 0.59583333 0.6 0.60416667 0.60833333 0.6125 0.61666667 0.62083333 0.625 0.62916667 0.63333333 0.6375 0.64166667 0.64583333 0.65 0.65416667 0.65833333 0.6625 0.66666667 0.67083333 0.675 0.67916667 0.68333333 0.6875 0.69166667 0.69583333 0.7 0.70416667 0.70833333 0.7125 0.71666667 0.72083333 0.725 0.72916667 0.73333333 0.7375 0.74166667 0.74583333 0.75 0.75416667 0.75833333 0.7625 0.76666667 0.77083333 0.775 0.77916667 0.78333333 0.7875 0.79166667 0.79583333 0.8 0.80416667 0.80833333 0.8125 0.81666667 0.82083333 0.825 0.82916667 0.83333333 0.8375 0.84166667 0.84583333 0.85 0.85416667 0.85833333 0.8625 0.86666667 0.87083333 0.875 0.87916667 0.88333333 0.8875 0.89166667 0.89583333 0.9 0.90416667 0.90833333 0.9125 0.91666667 0.92083333 0.925 0.92916667 0.93333333 0.9375 0.94166667 0.94583333 0.95 0.95416667 0.95833333 0.9625 0.96666667 0.97083333 0.975 0.97916667 0.98333333 0.9875 0.99166667 0.99583333 1 1 1 1 1 1
  arc A21 (6.1608, -15.8444) -> (6.8473, -15.56) centre (0, 0) ccw
  spline S21 degree 5 poles (6.8473, -15.56) (6.8475, -15.5572) (6.8479, -15.5517) (6.8485, -15.5433) (6.8492, -15.5322) (6.8502, -15.5184) (6.851, -15.5045) (6.8519, -15.4907) (6.8528, -15.477) (6.8536, -15.4632) (6.8544, -15.4495) (6.8551, -15.4358) (6.8559, -15.4222) (6.8566, -15.4086) (6.8573, -15.395) (6.8579, -15.3814) (6.8586, -15.3679) (6.8592, -15.3544) (6.8598, -15.341) (6.8603, -15.3275) (6.8609, -15.3141) (6.8614, -15.3008) (6.8619, -15.2874) (6.8623, -15.2741) (6.8628, -15.2609) (6.8632, -15.2476) (6.8636, -15.2344) (6.8639, -15.2213) (6.8642, -15.2081) (6.8646, -15.195) (6.8648, -15.182) (6.8651, -15.1689) (6.8653, -15.1559) (6.8656, -15.143) (6.8657, -15.13) (6.8659, -15.1171) (6.866, -15.1043) (6.8662, -15.0915) (6.8663, -15.0787) (6.8663, -15.0659) (6.8664, -15.0532) (6.8664, -15.0405) (6.8664, -15.0278) (6.8664, -15.0152) (6.8663, -15.0026) (6.8662, -14.9901) (6.8661, -14.9776) (6.866, -14.9651) (6.8659, -14.9527) (6.8657, -14.9403) (6.8655, -14.9279) (6.8653, -14.9156) (6.8651, -14.9033) (6.8649, -14.891) (6.8646, -14.8788) (6.8643, -14.8666) (6.864, -14.8545) (6.8636, -14.8424) (6.8633, -14.8303) (6.8629, -14.8183) (6.8625, -14.8063) (6.8621, -14.7943) (6.8616, -14.7824) (6.8611, -14.7705) (6.8606, -14.7587) (6.8601, -14.7469) (6.8596, -14.7351) (6.8591, -14.7234) (6.8585, -14.7117) (6.8579, -14.7001) (6.8573, -14.6885) (6.8567, -14.6769) (6.856, -14.6654) (6.8553, -14.6539) (6.8546, -14.6425) (6.8539, -14.6311) (6.8532, -14.6197) (6.8524, -14.6084) (6.8517, -14.5971) (6.8509, -14.5859) (6.8501, -14.5747) (6.8493, -14.5635) (6.8484, -14.5524) (6.8475, -14.5414) (6.8467, -14.5303) (6.8458, -14.5194) (6.8449, -14.5084) (6.8439, -14.4975) (6.843, -14.4867) (6.842, -14.4759) (6.841, -14.4651) (6.84, -14.4544) (6.839, -14.4437) (6.8379, -14.4331) (6.8369, -14.4225) (6.8358, -14.4119) (6.8347, -14.4014) (6.8336, -14.391) (6.8325, -14.3805) (6.8314, -14.3702) (6.8302, -14.3599) (6.829, -14.3496) (6.8278, -14.3394) (6.8266, -14.3292) (6.8254, -14.319) (6.8242, -14.309) (6.823, -14.2989) (6.8217, -14.2889) (6.8204, -14.279) (6.8191, -14.2691) (6.8178, -14.2592) (6.8165, -14.2494) (6.8152, -14.2397) (6.8138, -14.2299) (6.8125, -14.2203) (6.8111, -14.2107) (6.8097, -14.2011) (6.8083, -14.1916) (6.8069, -14.1821) (6.8055, -14.1727) (6.8041, -14.1634) (6.8026, -14.154) (6.8011, -14.1448) (6.7997, -14.1356) (6.7982, -14.1264) (6.7967, -14.1173) (6.7952, -14.1082) (6.7937, -14.0992) (6.7922, -14.0903) (6.7906, -14.0814) (6.7891, -14.0725) (6.7875, -14.0637) (6.786, -14.055) (6.7844, -14.0463) (6.7828, -14.0376) (6.7812, -14.0291) (6.7796, -14.0205) (6.778, -14.012) (6.7764, -14.0036) (6.7747, -13.9953) (6.7731, -13.9869) (6.7715, -13.9787) (6.7698, -13.9705) (6.7682, -13.9623) (6.7665, -13.9542) (6.7648, -13.9462) (6.7632, -13.9382) (6.7615, -13.9303) (6.7598, -13.9224) (6.7581, -13.9146) (6.7564, -13.9069) (6.7547, -13.8992) (6.753, -13.8916) (6.7513, -13.884) (6.7496, -13.8765) (6.7478, -13.869) (6.7461, -13.8616) (6.7444, -13.8543) (6.7427, -13.847) (6.7409, -13.8398) (6.7392, -13.8327) (6.7374, -13.8256) (6.7357, -13.8185) (6.734, -13.8116) (6.7322, -13.8047) (6.7305, -13.7978) (6.7287, -13.791) (6.727, -13.7843) (6.7253, -13.7777) (6.7235, -13.7711) (6.7218, -13.7645) (6.72, -13.7581) (6.7183, -13.7517) (6.7166, -13.7454) (6.7148, -13.7391) (6.7131, -13.7329) (6.7114, -13.7268) (6.7097, -13.7207) (6.7079, -13.7147) (6.7062, -13.7088) (6.7045, -13.7029) (6.7028, -13.6971) (6.7011, -13.6914) (6.6994, -13.6858) (6.6977, -13.6802) (6.6961, -13.6747) (6.6944, -13.6692) (6.6927, -13.6639) (6.6911, -13.6586) (6.6894, -13.6533) (6.6878, -13.6482) (6.6862, -13.6431) (6.6845, -13.6381) (6.6829, -13.6332) (6.6813, -13.6283) (6.6798, -13.6235) (6.6782, -13.6188) (6.6766, -13.6142) (6.6751, -13.6096) (6.6736, -13.6051) (6.672, -13.6007) (6.6705, -13.5964) (6.669, -13.5922) (6.6676, -13.588) (6.6661, -13.5839) (6.6647, -13.5799) (6.6633, -13.576) (6.6619, -13.5722) (6.6605, -13.5684) (6.6591, -13.5647) (6.6578, -13.5611) (6.6565, -13.5576) (6.6552, -13.5542) (6.6539, -13.5509) (6.6526, -13.5476) (6.6514, -13.5445) (6.6502, -13.5414) (6.649, -13.5384) (6.6479, -13.5355) (6.6468, -13.5327) (6.6457, -13.53) (6.6446, -13.5274) (6.6436, -13.5248) (6.6426, -13.5224) (6.6416, -13.5201) (6.6406, -13.5178) (6.6397, -13.5156) (6.6389, -13.5136) (6.638, -13.5116) (6.6372, -13.5098) (6.6364, -13.508) (6.6357, -13.5063) (6.635, -13.5048) (6.6344, -13.5033) (6.6338, -13.502) (6.6332, -13.5007) (6.6327, -13.4996) (6.6322, -13.4985) (6.6318, -13.4976) (6.6314, -13.4968) (6.6311, -13.4961) (6.6308, -13.4956) (6.6307, -13.4953) (6.6306, -13.4951) (6.6306, -13.495) knots -1 -1 -1 -1 -1 -1 -0.99583333 -0.99166667 -0.9875 -0.98333333 -0.97916667 -0.975 -0.97083333 -0.96666667 -0.9625 -0.95833333 -0.95416667 -0.95 -0.94583333 -0.94166667 -0.9375 -0.93333333 -0.92916667 -0.925 -0.92083333 -0.91666667 -0.9125 -0.90833333 -0.90416667 -0.9 -0.89583333 -0.89166667 -0.8875 -0.88333333 -0.87916667 -0.875 -0.87083333 -0.86666667 -0.8625 -0.85833333 -0.85416667 -0.85 -0.84583333 -0.84166667 -0.8375 -0.83333333 -0.82916667 -0.825 -0.82083333 -0.81666667 -0.8125 -0.80833333 -0.80416667 -0.8 -0.79583333 -0.79166667 -0.7875 -0.78333333 -0.77916667 -0.775 -0.77083333 -0.76666667 -0.7625 -0.75833333 -0.75416667 -0.75 -0.74583333 -0.74166667 -0.7375 -0.73333333 -0.72916667 -0.725 -0.72083333 -0.71666667 -0.7125 -0.70833333 -0.70416667 -0.7 -0.69583333 -0.69166667 -0.6875 -0.68333333 -0.67916667 -0.675 -0.67083333 -0.66666667 -0.6625 -0.65833333 -0.65416667 -0.65 -0.64583333 -0.64166667 -0.6375 -0.63333333 -0.62916667 -0.625 -0.62083333 -0.61666667 -0.6125 -0.60833333 -0.60416667 -0.6 -0.59583333 -0.59166667 -0.5875 -0.58333333 -0.57916667 -0.575 -0.57083333 -0.56666667 -0.5625 -0.55833333 -0.55416667 -0.55 -0.54583333 -0.54166667 -0.5375 -0.53333333 -0.52916667 -0.525 -0.52083333 -0.51666667 -0.5125 -0.50833333 -0.50416667 -0.5 -0.49583333 -0.49166667 -0.4875 -0.48333333 -0.47916667 -0.475 -0.47083333 -0.46666667 -0.4625 -0.45833333 -0.45416667 -0.45 -0.44583333 -0.44166667 -0.4375 -0.43333333 -0.42916667 -0.425 -0.42083333 -0.41666667 -0.4125 -0.40833333 -0.40416667 -0.4 -0.39583333 -0.39166667 -0.3875 -0.38333333 -0.37916667 -0.375 -0.37083333 -0.36666667 -0.3625 -0.35833333 -0.35416667 -0.35 -0.34583333 -0.34166667 -0.3375 -0.33333333 -0.32916667 -0.325 -0.32083333 -0.31666667 -0.3125 -0.30833333 -0.30416667 -0.3 -0.29583333 -0.29166667 -0.2875 -0.28333333 -0.27916667 -0.275 -0.27083333 -0.26666667 -0.2625 -0.25833333 -0.25416667 -0.25 -0.24583333 -0.24166667 -0.2375 -0.23333333 -0.22916667 -0.225 -0.22083333 -0.21666667 -0.2125 -0.20833333 -0.20416667 -0.2 -0.19583333 -0.19166667 -0.1875 -0.18333333 -0.17916667 -0.175 -0.17083333 -0.16666667 -0.1625 -0.15833333 -0.15416667 -0.15 -0.14583333 -0.14166667 -0.1375 -0.13333333 -0.12916667 -0.125 -0.12083333 -0.11666667 -0.1125 -0.10833333 -0.10416667 -0.1 -0.09583333 -0.09166667 -0.0875 -0.08333333 -0.07916667 -0.075 -0.07083333 -0.06666667 -0.0625 -0.05833333 -0.05416667 -0.05 -0.04583333 -0.04166667 -0.0375 -0.03333333 -0.02916667 -0.025 -0.02083333 -0.01666667 -0.0125 -0.00833333 -0.00416667 0 0 0 0 0 0
  line L42 (6.6306, -13.495) -> (6.6302, -13.4942)
  line L43 (6.6302, -13.4942) -> (6.5045, -13.2384)
  arc A22 (6.5045, -13.2384) -> (7.3936, -12.7631) centre (0, 0) ccw
  line L44 (7.3936, -12.7631) -> (7.5365, -13.0098)
  line L45 (7.5365, -13.0098) -> (7.537, -13.0105)